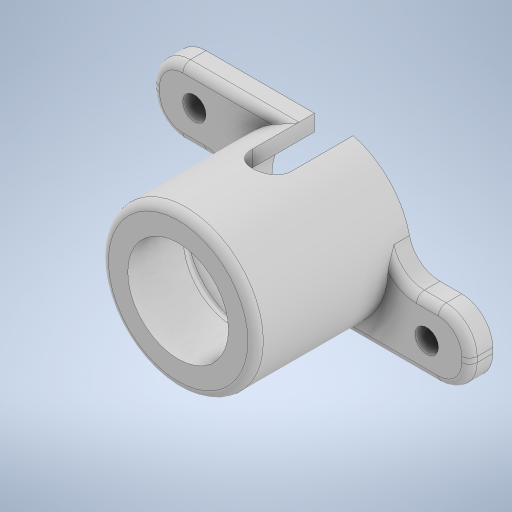
# Autodesk Inventor part: cover.ver1
Saved by Autodesk Inventor 2023 (Build 270158000, 158)
## iProperties
Created: 2023-11-07
Part Number: cover.ver1
Material: 一般
Document SubType Name: Modeling
Designer: bonju
Density: 1 g/cm^3
Appearance: 既定
Author: bonju
Autodesk Inventor part; units mm, degrees
ref_plane "YZ Plane" through (0, 0, 0) normal (1, 0, 0) x (0, 1, 0)
ref_plane "XZ Plane" through (0, 0, 0) normal (0, 1, 0) x (-1, 0, 0)
ref_plane "XY Plane" through (0, 0, 0) normal (0, 0, 1) x (1, 0, 0)
sketch "スケッチ1" plane through (0, 0, 0) normal (0, 0, 1) x (1, 0, 0)
  circle A0 centre (0, 0) radius 8
  circle A1 centre (0, 0) radius 10
  dimension "d0" = 16
  dimension "d1" = 2
  constraints: 2 centre point, 1 coincident
  measures "d0" diameter of A0
  measures "d1" radial gap between concentric circles of A0 A1
extrude "押し出し1" add sketch "スケッチ1" along normal blind 12
sketch "スケッチ2" plane through (0, 0, 12) normal (0, 0, 1) x (1, 0, 0)
  circle A0 centre (0, 0) radius 6.5
  circle A1 centre (0, 0) radius 10 projected
  circle A2 centre (0, 0) radius 10
  dimension "d4" = 13
  constraints: 2 centre point, 2 coincident
  measures "d4" diameter of A0
extrude "押し出し2" add sketch "スケッチ2" along normal blind 8.1
sketch "スケッチ3" plane through (0, 0, 0) normal (0, 1, 0) x (-1, 0, 0)
  line L0 (10, 0) -> (-10, 0) projected
  line L1 (2.5, 0) -> (2.5, 8)
  arc A0 (2.5, 8) -> (-2.5, 8) centre (0, 8) ccw
  line L2 (-2.5, 8) -> (-2.5, 0)
  line L3 (2.5, 0) -> (-2.5, 0)
  line L4 (0, -2.1) -> (0, 12.6) projected
  point P0 (0, 0)
  dimension "d7" = 5
  dimension "d8" = 8
  constraints: 6 end point, 2 point on circle, 2 point on line, 2 tangent, 1 centre point, 1 collinear, 1 parallel, 1 vertical, 1 other
  measures "d7" distance between parallel lines of L2 L1
  measures "d8" distance of L1.start L1.end
extrude "押し出し3" cut sketch "スケッチ3" along normal through all both and the other way through all
fillet "フィレット1" radius 1 2 edges at (-8, 0, 12) (-6.5, 0, 12)
fillet "フィレット2" radius 1 1 edges at (-10, 0, 20.1)
sketch "スケッチ4" plane through (0, 0, 0) normal (0, 0, -1) x (-1, 0, 0)
  line L0 (2.5, -9.682458) -> (2.5, -7.599342)
  line L1 (2.5, 9.682458) -> (20.5, 9.682458)
  line L2 (20.5, 9.682458) -> (20.5, 1)
  line L3 (2.5, 7.599342) -> (2.5, 9.682458)
  arc A0 (9.949874, 1) -> (2.5, 9.682458) centre (0, 0) ccw
  line L4 (0, -14) -> (0, 14)
  line L5 (20.5, 1) -> (9.949874, 1)
  arc A1 (2.5, -9.682458) -> (2.5, 9.682458) centre (0, 0) ccw
  line L6 (28.7, 0) -> (-28.7, 0)
  line L7 (2.5, 9.682458) -> (2.5, 7.599342)
  arc A2 (9.949874, 1) -> (2.5, 9.682458) centre (0, 0) ccw
  line L8 (-20.5, -1) -> (-9.949874, -1)
  arc A3 (-9.949874, -1) -> (-2.5, -9.682458) centre (0, 0) ccw
  line L9 (-2.5, -9.682458) -> (-20.5, -9.682458)
  line L10 (-20.5, -9.682458) -> (-20.5, -1)
  dimension "d22" = 1
  dimension "d23" = 20.5
  dimension "d26" = 360
  constraints: 12 end point, 7 point on circle, 3 centre point, 2 coincident, 2 horizontal, 1 perpendicular, 19 other
  measures "d22" distance between parallel lines of L6 L5
  measures "d23" distance from line of A1.centre L2
extrude "押し出し4" add sketch "スケッチ4" against normal blind 3
fillet "フィレット3" radius 4 4 edges at (-20.5, 9.6825, 1.5) (20.5, -9.6825, 1.5) (20.5, -1, 1.5) (-20.5, 1, 1.5)
fillet "フィレット3" radius 4 2 edges at (9.9499, -1, 1.5) (-9.9499, 1, 1.5)
fillet "フィレット4" radius 1 9 edges at (-19.3284, 8.5109, 3) (-9.5, 9.6825, 3) (-20.5, 5.3412, 3) (19.3284, -8.5109, 3) (20.5, -5.3412, 3) (19.3284, -2.1716, 3) (15.0874, -1, 3) (11.1677, -0.1168, 3) (9.5, -9.6825, 3)
sketch "スケッチ5" plane through (0, 0, 3) normal (0, 0, 1) x (1, 0, 0)
  circle A0 centre (0, 0) radius 10
  line L0 (-30.557695, 0) -> (39.846169, 0)
  line L1 (0, -14.002419) -> (0, 14.002419)
  line L2 (13.674794, -1) -> (20.5, -1)
  line L3 (20.5, -9.682458) -> (2.5, -9.682458)
  circle A1 centre (15, -5.5) radius 1.5
  line L4 (10, 9.263629) -> (10, 1.109348) construction
  circle A2 centre (-15, 5.5) radius 1.5
  line L5 (-28.7, 0) -> (28.7, 0)
  point P0 (9.949874, -1)
  point P1 (20.5, -5.341229)
  point P2 (20.5, -5.341229)
  dimension "d28" = 3
  dimension "d29" = 5
  dimension "d32" = 360
  dimension "d35" = 5.5
  constraints: 2 centre point, 2 end point, 1 parallel, 1 tangent, 1 vertical, 5 other
  measures "d28" diameter of A1
  measures "d29" distance from line of L4 A1.centre
  measures "d35" distance from line of A1.centre L5
extrude "押し出し5" cut sketch "スケッチ5" against normal through all contours A1 | A2
